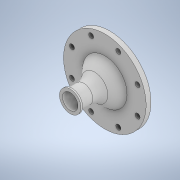
# Autodesk Inventor part: Крышка_быстроходного
Saved by Autodesk Inventor 2021 (Build 250183000, 183)
## iProperties
Created: 2023-03-23
Part Number: Крышка_быстроходного
Material: Типовые
Document SubType Name: Modeling
Designer: gdevc
Density: 1 g/cm^3
Appearance: По умолчанию
Mass: 638.282 g
Surface Area: 1460.85 cm^2
Volume: 638.282 cm^3
Author: gdevc
Autodesk Inventor part; units mm, degrees
ref_plane "YZ Plane" through (0, 0, 0) normal (1, 0, 0) x (0, 1, 0)
ref_plane "XZ Plane" through (0, 0, 0) normal (0, 1, 0) x (-1, 0, 0)
ref_plane "XY Plane" through (0, 0, 0) normal (0, 0, 1) x (1, 0, 0)
sketch "Эскиз1" plane through (0, 0, 0) normal (1, 0, 0) x (0, 1, 0)
  line L0 (0, 0) -> (0, -73.7994) construction
  line L1 (23.5, 0) -> (23.5, -65.8206)
  line L2 (23.5, -65.8206) -> (67.6779, -115.777)
  line L3 (125, -110.9688) -> (125, -104.777)
  line L4 (125, -104.777) -> (67.2948, -104.777)
  line L5 (67.2948, -104.777) -> (40.0448, -73.9627)
  line L6 (27.5, -40.8401) -> (27.5, -5)
  line L7 (27.5, -5) -> (32.5, -5)
  line L8 (32.5, -5) -> (32.5, 0)
  line L9 (32.5, 0) -> (23.5, 0)
  line L10 (67.6779, -115.777) -> (90, -115.777)
  line L11 (90, -115.777) -> (90, -119.777)
  line L12 (90, -119.777) -> (125, -119.777)
  line L13 (125, -119.777) -> (125, -110.9688)
  arc A0 (27.5, -40.8401) -> (40.0448, -73.9627) centre (77.5, -40.8401) ccw
  point P0 (27.5, -59.777)
  point P1 (125, -98)
  dimension "d13" = 47
  dimension "d14" = 180
  dimension "d15" = 250
  dimension "d16" = 7
  dimension "d18" = 0
  dimension "d19" = 15
  dimension "d20" = 4
  dimension "d21" = 65
  dimension "d22" = 4
  dimension "d23" = 5
  dimension "d24" = 59.777
  dimension "d25" = 60
  dimension "d53" = 50
  constraints: 28 end point, 7 perpendicular, 2 parallel, 2 point on circle, 2 point on line, 2 tangent, 2 vertical, 1 centre point, 1 horizontal
  measures "d13" diameter of L1 L0
  measures "d14" diameter of L11 L0
  measures "d15" diameter of L13 L0
  measures "d16" distance between parallel lines of L2 L5
  measures "d18" distance from line of L0.start L9
  measures "d19" distance between parallel lines of L12 L4
  measures "d20" distance of L10.end L11.end
  measures "d21" diameter of L8 L0
  measures "d22" distance between parallel lines of L1 L6
  measures "d23" distance between parallel lines of L9 L7
  measures "d24" vertical distance of L0.start point (27.5, -59.777)
  measures "d25" distance from line of L12 point (27.5, -59.777)
  measures "d53" radius of A0
revolve "Вращение1" add sketch "Эскиз1" angle 360 about axis through (0, 0, 0) along (0, 0, -1)
sketch "Эскиз2" plane through (0, 0, -119.777) normal (0, 0, -1) x (-1, 0, 0)
  circle A0 centre (-41.139, 99.317) radius 7.5
  circle A1 centre (0, 0) radius 107.5
  circle A2 centre (-99.3174, 41.1381) radius 7.5
  circle A3 centre (-99.317, -41.139) radius 7.5
  circle A4 centre (-41.1381, -99.3174) radius 7.5
  circle A5 centre (41.139, -99.317) radius 7.5
  circle A6 centre (99.3174, -41.1381) radius 7.5
  circle A7 centre (99.317, 41.139) radius 7.5
  circle A8 centre (41.1381, 99.3174) radius 7.5
  dimension "d27" = 215
  dimension "d28" = 15
  dimension "d29" = 41.139
  dimension "d30" = 99.317
  dimension "d33" = 360
  constraints: 9 centre point, 1 coincident, 17 other
  measures "d27" diameter of A1
  measures "d28" diameter of A0
  measures "d29" horizontal distance of point (0, 0) A0.centre
  measures "d30" vertical distance of point (0, 0) A0.centre
extrude "Выдавливание1" cut sketch "Эскиз2" against normal through all contours A0 A1 | A1 A0 | A8 A1 | A1 A8 | A2 A1 | A1 A2 | A7 A1 | A1 A7 | A3 A1 | A1 A3 | A4 A1 | A1 A4 | A6 A1 | A1 A6 | A5 A1 | A1 A5
thread "Резьба1" size "M15x1.5" class "6H" standard "ISO Metric profile" length 18
thread "Резьба2" size "M15x1.5" class "6H" standard "ISO Metric profile" length 18
thread "Резьба3" size "M15x1.5" class "6H" standard "ISO Metric profile" length 18
thread "Резьба4" size "M15x1.5" class "6H" standard "ISO Metric profile" length 18
thread "Резьба5" size "M15x1.5" class "6H" standard "ISO Metric profile" length 18
thread "Резьба6" size "M15x1.5" class "6H" standard "ISO Metric profile" length 18
thread "Резьба7" size "M15x1.5" class "6H" standard "ISO Metric profile" length 18
thread "Резьба8" size "M15x1.5" class "6H" standard "ISO Metric profile" length 18
